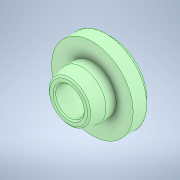
# Autodesk Inventor part: encoder_codewheel_pwb_mount
Saved by Autodesk Inventor 2022.2 (Build 262287000, 287)
## iProperties
Created: 2019-07-04
Part Number: encoder_codewheel_pwb_mount
Material: Generic
Document SubType Name: Modeling
Designer: Jochen
Density: 1 g/cm^3
Appearance: Default
Sending System: SolidWorks 2017
Last Author: Felix
Last Saved: 2021-02-23
Author: Jochen
Autodesk Inventor part; units mm, degrees
ref_plane "YZ Plane" through (0, 0, 0) normal (1, 0, 0) x (0, 1, 0)
ref_plane "XZ Plane" through (0, 0, 0) normal (0, 1, 0) x (-1, 0, 0)
ref_plane "Work Plane3" through (0, 0, 15) normal (0, 0, 1) x (1, 0, 0)
sketch "Sketch1" plane through (0, 0, 15) normal (0, 0, 1) x (1, 0, 0)
  line L0 (-8.4, 0) -> (8.4, 0) construction
  line L1 (0, -8.4) -> (0, 8.4) construction
  circle A0 centre (0, 0) radius 2.1
  circle A1 centre (0, 0) radius 3.5
  circle A2 centre (0, 0) radius 6
  arc A3 (0.3976, 3.7246) -> (0.5788, 3.8401) centre (0.3976, 3.9246) ccw
  line L2 (0.5788, 3.8401) -> (0.7363, 4.1779)
  arc A4 (1.0807, 4.3422) -> (0.7363, 4.1779) centre (1.0082, 4.0511) ccw
  arc A5 (1.2352, 4.3008) -> (1.0807, 4.3422) centre (0, 0) ccw
  arc A6 (1.4512, 3.9863) -> (1.2352, 4.3008) centre (1.1524, 4.0124) ccw
  line L3 (1.4512, 3.9863) -> (1.4188, 3.6151)
  arc A7 (1.4188, 3.6151) -> (1.518, 3.4244) centre (1.618, 3.5976) ccw
  line L4 (1.518, 3.4244) -> (2.2066, 3.0268)
  arc A8 (2.2066, 3.0268) -> (2.4214, 3.0362) centre (2.3066, 3.2001) ccw
  line L5 (2.4214, 3.0362) -> (2.7266, 3.25)
  arc A9 (3.107, 3.2201) -> (2.7266, 3.25) centre (2.8987, 3.0042) ccw
  arc A10 (3.2201, 3.107) -> (3.107, 3.2201) centre (0, 0) ccw
  arc A11 (3.25, 2.7266) -> (3.2201, 3.107) centre (3.0042, 2.8987) ccw
  line L6 (3.25, 2.7266) -> (3.0362, 2.4214)
  arc A12 (3.0362, 2.4214) -> (3.0268, 2.2066) centre (3.2001, 2.3066) ccw
  line L7 (3.0268, 2.2066) -> (3.4244, 1.518)
  arc A13 (3.4244, 1.518) -> (3.6151, 1.4188) centre (3.5976, 1.618) ccw
  line L8 (3.6151, 1.4188) -> (3.9863, 1.4512)
  arc A14 (4.3008, 1.2352) -> (3.9863, 1.4512) centre (4.0124, 1.1524) ccw
  arc A15 (4.3422, 1.0807) -> (4.3008, 1.2352) centre (0, 0) ccw
  arc A16 (4.1779, 0.7363) -> (4.3422, 1.0807) centre (4.0511, 1.0082) ccw
  line L9 (4.1779, 0.7363) -> (3.8401, 0.5788)
  arc A17 (3.8401, 0.5788) -> (3.7246, 0.3976) centre (3.9246, 0.3976) ccw
  line L10 (3.7246, 0.3976) -> (3.7246, -0.3976)
  arc A18 (3.7246, -0.3976) -> (3.8401, -0.5788) centre (3.9246, -0.3976) ccw
  line L11 (3.8401, -0.5788) -> (4.1779, -0.7363)
  arc A19 (4.3422, -1.0807) -> (4.1779, -0.7363) centre (4.0511, -1.0082) ccw
  arc A20 (4.3008, -1.2352) -> (4.3422, -1.0807) centre (0, 0) ccw
  arc A21 (3.9863, -1.4512) -> (4.3008, -1.2352) centre (4.0124, -1.1524) ccw
  line L12 (3.9863, -1.4512) -> (3.6151, -1.4188)
  arc A22 (3.6151, -1.4188) -> (3.4244, -1.518) centre (3.5976, -1.618) ccw
  line L13 (3.4244, -1.518) -> (3.0268, -2.2066)
  arc A23 (3.0268, -2.2066) -> (3.0362, -2.4214) centre (3.2001, -2.3066) ccw
  line L14 (3.0362, -2.4214) -> (3.25, -2.7266)
  arc A24 (3.2201, -3.107) -> (3.25, -2.7266) centre (3.0042, -2.8987) ccw
  arc A25 (3.107, -3.2201) -> (3.2201, -3.107) centre (0, 0) ccw
  arc A26 (2.7266, -3.25) -> (3.107, -3.2201) centre (2.8987, -3.0042) ccw
  line L15 (2.7266, -3.25) -> (2.4214, -3.0362) construction
  arc A27 (2.4214, -3.0362) -> (2.2066, -3.0268) centre (2.3066, -3.2001) ccw construction
  line L16 (2.2066, -3.0268) -> (1.518, -3.4244) construction
  arc A28 (1.518, -3.4244) -> (1.4188, -3.6151) centre (1.618, -3.5976) ccw construction
  line L17 (1.4188, -3.6151) -> (1.4512, -3.9863) construction
  arc A29 (1.2352, -4.3008) -> (1.4512, -3.9863) centre (1.1524, -4.0124) ccw construction
  arc A30 (1.0807, -4.3422) -> (1.2352, -4.3008) centre (0, 0) ccw construction
  arc A31 (0.7363, -4.1779) -> (1.0807, -4.3422) centre (1.0082, -4.0511) ccw construction
  line L18 (0.7363, -4.1779) -> (0.5788, -3.8401) construction
  arc A32 (0.5788, -3.8401) -> (0.3976, -3.7246) centre (0.3976, -3.9246) ccw construction
  line L19 (0.3976, -3.7246) -> (-0.3976, -3.7246) construction
  arc A33 (-0.3976, -3.7246) -> (-0.5788, -3.8401) centre (-0.3976, -3.9246) ccw construction
  line L20 (-0.5788, -3.8401) -> (-0.7363, -4.1779) construction
  arc A34 (-1.0807, -4.3422) -> (-0.7363, -4.1779) centre (-1.0082, -4.0511) ccw construction
  arc A35 (-1.2352, -4.3008) -> (-1.0807, -4.3422) centre (0, 0) ccw construction
  arc A36 (-1.4512, -3.9863) -> (-1.2352, -4.3008) centre (-1.1524, -4.0124) ccw construction
  line L21 (-1.4512, -3.9863) -> (-1.4188, -3.6151) construction
  arc A37 (-1.4188, -3.6151) -> (-1.518, -3.4244) centre (-1.618, -3.5976) ccw construction
  line L22 (-1.518, -3.4244) -> (-2.2066, -3.0268) construction
  arc A38 (-2.2066, -3.0268) -> (-2.4214, -3.0362) centre (-2.3066, -3.2001) ccw construction
  line L23 (-2.4214, -3.0362) -> (-2.7266, -3.25) construction
  arc A39 (-3.107, -3.2201) -> (-2.7266, -3.25) centre (-2.8987, -3.0042) ccw construction
  arc A40 (-3.2201, -3.107) -> (-3.107, -3.2201) centre (0, 0) ccw construction
  arc A41 (-3.25, -2.7266) -> (-3.2201, -3.107) centre (-3.0042, -2.8987) ccw construction
  line L24 (-3.25, -2.7266) -> (-3.0362, -2.4214) construction
  arc A42 (-3.0362, -2.4214) -> (-3.0268, -2.2066) centre (-3.2001, -2.3066) ccw construction
  line L25 (-3.0268, -2.2066) -> (-3.4244, -1.518) construction
  arc A43 (-3.4244, -1.518) -> (-3.6151, -1.4188) centre (-3.5976, -1.618) ccw construction
  line L26 (-3.6151, -1.4188) -> (-3.9863, -1.4512) construction
  arc A44 (-4.3008, -1.2352) -> (-3.9863, -1.4512) centre (-4.0124, -1.1524) ccw construction
  arc A45 (-4.3422, -1.0807) -> (-4.3008, -1.2352) centre (0, 0) ccw construction
  arc A46 (-4.1779, -0.7363) -> (-4.3422, -1.0807) centre (-4.0511, -1.0082) ccw construction
  line L27 (-4.1779, -0.7363) -> (-3.8401, -0.5788) construction
  arc A47 (-3.8401, -0.5788) -> (-3.7246, -0.3976) centre (-3.9246, -0.3976) ccw construction
  line L28 (-3.7246, -0.3976) -> (-3.7246, 0.3976) construction
  arc A48 (-3.7246, 0.3976) -> (-3.8401, 0.5788) centre (-3.9246, 0.3976) ccw construction
  line L29 (-3.8401, 0.5788) -> (-4.1779, 0.7363) construction
  arc A49 (-4.3422, 1.0807) -> (-4.1779, 0.7363) centre (-4.0511, 1.0082) ccw construction
  arc A50 (-4.3008, 1.2352) -> (-4.3422, 1.0807) centre (0, 0) ccw construction
  arc A51 (-3.9863, 1.4512) -> (-4.3008, 1.2352) centre (-4.0124, 1.1524) ccw construction
  line L30 (-3.9863, 1.4512) -> (-3.6151, 1.4188) construction
  arc A52 (-3.6151, 1.4188) -> (-3.4244, 1.518) centre (-3.5976, 1.618) ccw construction
  line L31 (-3.4244, 1.518) -> (-3.0268, 2.2066) construction
  arc A53 (-3.0268, 2.2066) -> (-3.0362, 2.4214) centre (-3.2001, 2.3066) ccw construction
  line L32 (-3.0362, 2.4214) -> (-3.25, 2.7266) construction
  arc A54 (-3.2201, 3.107) -> (-3.25, 2.7266) centre (-3.0042, 2.8987) ccw construction
  arc A55 (-3.107, 3.2201) -> (-3.2201, 3.107) centre (0, 0) ccw construction
  arc A56 (-2.7266, 3.25) -> (-3.107, 3.2201) centre (-2.8987, 3.0042) ccw construction
  line L33 (-2.7266, 3.25) -> (-2.4214, 3.0362)
  arc A57 (-2.4214, 3.0362) -> (-2.2066, 3.0268) centre (-2.3066, 3.2001) ccw
  line L34 (-2.2066, 3.0268) -> (-1.518, 3.4244)
  arc A58 (-1.518, 3.4244) -> (-1.4188, 3.6151) centre (-1.618, 3.5976) ccw
  line L35 (-1.4188, 3.6151) -> (-1.4512, 3.9863)
  arc A59 (-1.2352, 4.3008) -> (-1.4512, 3.9863) centre (-1.1524, 4.0124) ccw
  arc A60 (-1.0807, 4.3422) -> (-1.2352, 4.3008) centre (0, 0) ccw
  arc A61 (-0.7363, 4.1779) -> (-1.0807, 4.3422) centre (-1.0082, 4.0511) ccw
  line L36 (-0.7363, 4.1779) -> (-0.5788, 3.8401)
  arc A62 (-0.5788, 3.8401) -> (-0.3976, 3.7246) centre (-0.3976, 3.9246) ccw
  line L37 (-0.3976, 3.7246) -> (0.3976, 3.7246)
  line L38 (-3.9776, -1.5509) -> (-3.6064, -1.5184)
  arc A63 (-3.511, -1.568) -> (-3.6064, -1.5184) centre (-3.5976, -1.618) ccw
  line L39 (-3.511, -1.568) -> (-3.1134, -2.2566)
  arc A64 (-3.1181, -2.364) -> (-3.1134, -2.2566) centre (-3.2001, -2.3066) ccw
  line L40 (-3.1181, -2.364) -> (-3.3319, -2.6693)
  arc A65 (-3.3319, -2.6693) -> (-3.2921, -3.1764) centre (-3.0042, -2.8987) ccw
  arc A66 (-3.2921, -3.1764) -> (-3.1764, -3.2921) centre (0, 0) ccw
  arc A67 (-3.1764, -3.2921) -> (-2.6693, -3.3319) centre (-2.8987, -3.0042) ccw
  line L41 (-2.6693, -3.3319) -> (-2.364, -3.1181)
  arc A68 (-2.2566, -3.1134) -> (-2.364, -3.1181) centre (-2.3066, -3.2001) ccw
  line L42 (-2.2566, -3.1134) -> (-1.568, -3.511)
  arc A69 (-1.5184, -3.6064) -> (-1.568, -3.511) centre (-1.618, -3.5976) ccw
  line L43 (-1.5184, -3.6064) -> (-1.5509, -3.9776)
  arc A70 (-1.5509, -3.9776) -> (-1.2628, -4.3969) centre (-1.1524, -4.0124) ccw
  arc A71 (-1.2628, -4.3969) -> (-1.1048, -4.4392) centre (0, 0) ccw
  arc A72 (-1.1048, -4.4392) -> (-0.6457, -4.2201) centre (-1.0082, -4.0511) ccw
  line L44 (-0.6457, -4.2201) -> (-0.4882, -3.8824)
  arc A73 (-0.3976, -3.8246) -> (-0.4882, -3.8824) centre (-0.3976, -3.9246) ccw
  line L45 (-0.3976, -3.8246) -> (0.3976, -3.8246)
  arc A74 (0.4882, -3.8824) -> (0.3976, -3.8246) centre (0.3976, -3.9246) ccw
  line L46 (0.4882, -3.8824) -> (0.6457, -4.2201)
  arc A75 (0.6457, -4.2201) -> (1.1048, -4.4392) centre (1.0082, -4.0511) ccw
  arc A76 (1.1048, -4.4392) -> (1.2628, -4.3969) centre (0, 0) ccw
  arc A77 (1.2628, -4.3969) -> (1.5509, -3.9776) centre (1.1524, -4.0124) ccw
  line L47 (1.5509, -3.9776) -> (1.5184, -3.6064)
  arc A78 (1.568, -3.511) -> (1.5184, -3.6064) centre (1.618, -3.5976) ccw
  line L48 (1.568, -3.511) -> (2.2566, -3.1134)
  arc A79 (2.364, -3.1181) -> (2.2566, -3.1134) centre (2.3066, -3.2001) ccw
  line L49 (2.364, -3.1181) -> (2.6693, -3.3319)
  arc A80 (2.6693, -3.3319) -> (3.1764, -3.2921) centre (2.8987, -3.0042) ccw
  arc A81 (3.1764, -3.2921) -> (3.2921, -3.1764) centre (0, 0) ccw
  arc A82 (3.2921, -3.1764) -> (3.3319, -2.6693) centre (3.0042, -2.8987) ccw
  line L50 (3.3319, -2.6693) -> (3.1181, -2.364)
  arc A83 (3.1134, -2.2566) -> (3.1181, -2.364) centre (3.2001, -2.3066) ccw
  line L51 (3.1134, -2.2566) -> (3.511, -1.568)
  arc A84 (3.6064, -1.5184) -> (3.511, -1.568) centre (3.5976, -1.618) ccw
  line L52 (3.6064, -1.5184) -> (3.9776, -1.5509)
  arc A85 (3.9776, -1.5509) -> (4.3969, -1.2628) centre (4.0124, -1.1524) ccw
  arc A86 (4.3969, -1.2628) -> (4.4392, -1.1048) centre (0, 0) ccw
  arc A87 (4.4392, -1.1048) -> (4.2201, -0.6457) centre (4.0511, -1.0082) ccw
  line L53 (4.2201, -0.6457) -> (3.8824, -0.4882)
  arc A88 (3.8246, -0.3976) -> (3.8824, -0.4882) centre (3.9246, -0.3976) ccw
  line L54 (3.8246, -0.3976) -> (3.8246, 0.3976)
  arc A89 (3.8824, 0.4882) -> (3.8246, 0.3976) centre (3.9246, 0.3976) ccw
  line L55 (3.8824, 0.4882) -> (4.2201, 0.6457)
  arc A90 (4.2201, 0.6457) -> (4.4392, 1.1048) centre (4.0511, 1.0082) ccw
  arc A91 (4.4392, 1.1048) -> (4.3969, 1.2628) centre (0, 0) ccw
  arc A92 (4.3969, 1.2628) -> (3.9776, 1.5509) centre (4.0124, 1.1524) ccw
  line L56 (3.9776, 1.5509) -> (3.6064, 1.5184)
  arc A93 (3.511, 1.568) -> (3.6064, 1.5184) centre (3.5976, 1.618) ccw
  line L57 (3.511, 1.568) -> (3.1134, 2.2566)
  arc A94 (3.1181, 2.364) -> (3.1134, 2.2566) centre (3.2001, 2.3066) ccw
  line L58 (3.1181, 2.364) -> (3.3319, 2.6693)
  arc A95 (3.3319, 2.6693) -> (3.2921, 3.1764) centre (3.0042, 2.8987) ccw
  arc A96 (3.2921, 3.1764) -> (3.1764, 3.2921) centre (0, 0) ccw
  arc A97 (3.1764, 3.2921) -> (2.6693, 3.3319) centre (2.8987, 3.0042) ccw
  line L59 (2.6693, 3.3319) -> (2.364, 3.1181)
  arc A98 (2.2566, 3.1134) -> (2.364, 3.1181) centre (2.3066, 3.2001) ccw
  line L60 (2.2566, 3.1134) -> (1.568, 3.511)
  arc A99 (1.5184, 3.6064) -> (1.568, 3.511) centre (1.618, 3.5976) ccw
  line L61 (1.5184, 3.6064) -> (1.5509, 3.9776)
  arc A100 (1.5509, 3.9776) -> (1.2628, 4.3969) centre (1.1524, 4.0124) ccw
  arc A101 (1.2628, 4.3969) -> (1.1048, 4.4392) centre (0, 0) ccw
  arc A102 (1.1048, 4.4392) -> (0.6457, 4.2201) centre (1.0082, 4.0511) ccw
  line L62 (0.6457, 4.2201) -> (0.4882, 3.8824)
  arc A103 (0.3976, 3.8246) -> (0.4882, 3.8824) centre (0.3976, 3.9246) ccw
  line L63 (0.3976, 3.8246) -> (-0.3976, 3.8246)
  arc A104 (-0.4882, 3.8824) -> (-0.3976, 3.8246) centre (-0.3976, 3.9246) ccw
  line L64 (-0.4882, 3.8824) -> (-0.6457, 4.2201)
  arc A105 (-0.6457, 4.2201) -> (-1.1048, 4.4392) centre (-1.0082, 4.0511) ccw
  arc A106 (-1.1048, 4.4392) -> (-1.2628, 4.3969) centre (0, 0) ccw
  arc A107 (-1.2628, 4.3969) -> (-1.5509, 3.9776) centre (-1.1524, 4.0124) ccw
  line L65 (-1.5509, 3.9776) -> (-1.5184, 3.6064)
  arc A108 (-1.568, 3.511) -> (-1.5184, 3.6064) centre (-1.618, 3.5976) ccw
  line L66 (-1.568, 3.511) -> (-2.2566, 3.1134)
  arc A109 (-2.364, 3.1181) -> (-2.2566, 3.1134) centre (-2.3066, 3.2001) ccw
  line L67 (-2.364, 3.1181) -> (-2.6693, 3.3319)
  arc A110 (-2.6693, 3.3319) -> (-3.1764, 3.2921) centre (-2.8987, 3.0042) ccw
  arc A111 (-3.1764, 3.2921) -> (-3.2921, 3.1764) centre (0, 0) ccw
  arc A112 (-3.2921, 3.1764) -> (-3.3319, 2.6693) centre (-3.0042, 2.8987) ccw
  line L68 (-3.3319, 2.6693) -> (-3.1181, 2.364)
  arc A113 (-3.1134, 2.2566) -> (-3.1181, 2.364) centre (-3.2001, 2.3066) ccw
  line L69 (-3.1134, 2.2566) -> (-3.511, 1.568)
  arc A114 (-3.6064, 1.5184) -> (-3.511, 1.568) centre (-3.5976, 1.618) ccw
  line L70 (-3.6064, 1.5184) -> (-3.9776, 1.5509)
  arc A115 (-3.9776, 1.5509) -> (-4.3969, 1.2628) centre (-4.0124, 1.1524) ccw
  arc A116 (-4.3969, 1.2628) -> (-4.4392, 1.1048) centre (0, 0) ccw
  arc A117 (-4.4392, 1.1048) -> (-4.2201, 0.6457) centre (-4.0511, 1.0082) ccw
  line L71 (-4.2201, 0.6457) -> (-3.8824, 0.4882)
  arc A118 (-3.8246, 0.3976) -> (-3.8824, 0.4882) centre (-3.9246, 0.3976) ccw
  line L72 (-3.8246, 0.3976) -> (-3.8246, -0.3976)
  arc A119 (-3.8824, -0.4882) -> (-3.8246, -0.3976) centre (-3.9246, -0.3976) ccw
  line L73 (-3.8824, -0.4882) -> (-4.2201, -0.6457)
  arc A120 (-4.2201, -0.6457) -> (-4.4392, -1.1048) centre (-4.0511, -1.0082) ccw
  arc A121 (-4.4392, -1.1048) -> (-4.3969, -1.2628) centre (0, 0) ccw
  arc A122 (-4.3969, -1.2628) -> (-3.9776, -1.5509) centre (-4.0124, -1.1524) ccw
  circle A123 centre (0, 0) radius 3.7246 construction
  point P0 (-3.2256, -1.8623)
  point P1 (-1.8623, -3.2256)
  point P2 (0, -3.7246)
  point P3 (1.8623, -3.2256)
  point P4 (3.2256, -1.8623)
  point P5 (3.7246, 0)
  point P6 (3.2256, 1.8623)
  point P7 (1.8623, 3.2256)
  point P8 (0, 3.7246)
  point P9 (-1.8623, 3.2256)
  point P10 (-3.2256, 1.8623)
  dimension "d3" = 4.2
  dimension "d4" = 7
  dimension "d5" = 12
  dimension "d29" = 0.1
  dimension "d30" = 0.7952
  dimension "d31" = 0.2
  dimension "d32" = 0.3726
  dimension "d33" = 0.3
  dimension "d34" = 4.4746
  constraints: 240 point on circle, 144 end point, 123 centre point, 23 equal radius, 18 equal length, 11 midpoint, 10 tangent, 4 coincident, 108 other
  measures "d3" diameter of A0
  measures "d4" diameter of A1
  measures "d5" diameter of A2
  measures "d29" radial gap between concentric circles of A44 A122
  measures "d30" distance of L28.start L28.end
  measures "d31" radius of A47
  measures "d32" distance of L27.start L27.end
  measures "d33" radius of A46
  measures "d34" radius of A45
extrude "Extrusion1" add sketch "Sketch1" against normal blind 3.5 contours A1
extrude "Extrusion2" add sketch "Sketch1" against normal blind 2 from surface at -3.5 contours A1 | A2 | A122 A121 A120 L73 A119 L72 A118 L71 A117 A116 A115 L70 A114 L69 A113 L68 A112 A111 A110 L67 A109 L66 A108 L65 A107 A106 A105 L64 A104 L63 A103 L62 A102 A101 A100 L61 A99 L60 A98 L59 A97 A96 A95 L58 A94 L57 A93 L56 A92 A91 A90 L55 A89 L54 A88 L53 A87 A86 A85 L52 A84 L51 A83 L50 A82 A81 A80 L49 A79 L48 A78 L47 A77 A76 A75 L46 A74 L45 A73 L44 A72 A71 A70 L43 A69 L42 A68 L41 A67 A66 A65 L40 A64 L39 A63 L38
extrude "Extrusion4" add sketch "Sketch1" against normal blind 0.8 from surface at -5.5 separate body contours A2
chamfer "Chamfer1" distance 0.8 angle 45 1 edges at (-6, 0, 8.7)
fillet "Fillet1" radius 0.2 1 edges at (-5.2001, 0, 8.7)
chamfer "Chamfer2" distance 0.2 distance2 0.8 1 edges at (-2.1, 0, 9.5) measured on face at (-2.6, 0, 9.5)
chamfer "Chamfer3" distance 0.5 distance2 2 1 edges at (-3.5, 0, 15) measured on face at (-3, 0, 15)
chamfer "Chamfer4" distance 0.2 angle 45 3 edges at (-3, 0, 15) (-2.1, 0, 15) (-2.3, 0, 9.5)
body "Solid1"
body "Solid2"
body "Solid3"
